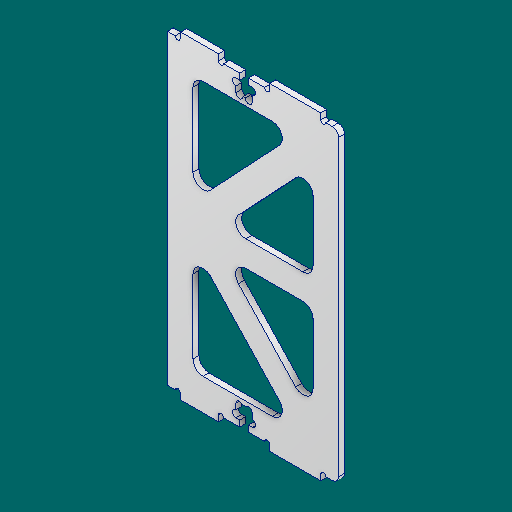
# Autodesk Inventor part: IntakeRamp
Saved by Autodesk Inventor 2023.1 (Build 271208000, 208)
## iProperties
Created: 2022-11-11
Part Number: IntakeRamp
Material: Aluminum 6061
Document SubType Name: Modeling
Designer: zac-h
Density: 2.7 g/cm^3
Appearance: Aluminum - Flat
Mass: 67.9744 g
Surface Area: 202.14 cm^2
Volume: 25.1757 cm^3
Author: zac-h
Autodesk Inventor part; units mm, degrees
ref_plane "YZ Plane" through (0, 0, 0) normal (1, 0, 0) x (0, 1, 0)
ref_plane "XZ Plane" through (0, 0, 0) normal (0, 1, 0) x (-1, 0, 0)
ref_plane "XY Plane" through (0, 0, 0) normal (0, 0, 1) x (1, 0, 0)
sketch "Sketch1" plane through (0, 0, 0) normal (0, 0, 1) x (1, 0, 0)
  line L0 (0, 0) -> (18.773541, 0)
  line L1 (18.773541, 0) -> (18.773541, 3)
  line L2 (-0.276459, 3) -> (18.773541, 3) construction
  line L3 (-0.276459, 0) -> (-0.276459, 3)
  line L4 (29.314541, 3) -> (33.632541, 3) construction
  line L5 (44.173541, 0) -> (69.573541, 0)
  line L6 (69.573541, 0) -> (69.573541, 3)
  line L7 (44.173541, 3) -> (69.573541, 3) construction
  line L8 (44.173541, 0) -> (44.173541, 3)
  line L9 (-0.276459, 3) -> (-6.626459, 3)
  line L10 (-0.276459, 3) -> (6.073541, 3) construction
  line L11 (-6.626459, 3) -> (-6.626459, 79.2)
  line L12 (-6.626459, 79.2) -> (78.463541, 79.2)
  line L13 (69.573541, 3) -> (78.463541, 3)
  line L14 (78.463541, 3) -> (78.463541, 79.2)
  line L15 (18.773541, 3) -> (29.314541, 3)
  line L16 (44.173541, 3) -> (33.632541, 3)
  line L17 (33.632541, 3) -> (33.632541, 6)
  line L18 (33.632541, 6) -> (35.537541, 6)
  line L19 (35.537541, 6) -> (35.537541, 12.35)
  line L20 (35.537541, 12.35) -> (27.409541, 12.35)
  line L21 (27.409541, 12.35) -> (27.409541, 6)
  line L22 (27.409541, 6) -> (29.314541, 6)
  line L23 (29.314541, 6) -> (29.314541, 3)
  circle A0 centre (20.023541, 3) radius 1.25
  circle A1 centre (-1.526459, 3) radius 1.25
  circle A2 centre (42.923541, 3) radius 1.25
  circle A3 centre (70.823541, 3) radius 1.25
  circle A4 centre (35.537541, 7.75) radius 1.75
  circle A5 centre (27.409541, 7.75) radius 1.75
  circle A6 centre (33.787541, 12.35) radius 1.75
  circle A7 centre (29.159541, 12.35) radius 1.75
  point P0 (28.362041, 6)
  point P1 (21.273541, 3)
  point P2 (27.409541, 9.5)
  point P3 (30.909541, 12.35)
  point P4 (32.037541, 12.35)
  point P5 (35.537541, 9.5)
  point P6 (41.673541, 3)
  point P7 (72.073541, 3)
  point P8 (-2.776459, 3)
  dimension "d9" = 2.5
  dimension "d10" = 3.5
  dimension "d11" = 3.5
  dimension "d0" = 6.35
  dimension "d1" = 180
  dimension "d2" = 76.2
  dimension "d3" = 8.89
  dimension "d4" = 3
  dimension "d5" = 8.128
  dimension "d6" = 6.35
  constraints: 30 end point, 10 point on line, 6 perpendicular, 5 horizontal, 3 collinear, 2 vertical, 1 midpoint, 1 parallel, 24 other
  measures "d0" distance of L2.start L9.end
  measures "d1" angle of L9 L10
  measures "d2" distance of L9.end L11.end
  measures "d3" distance of L6.end L13.end
  measures "d4" distance of L4.end L17.end
  measures "d5" distance between parallel lines of L19 L21
  measures "d6" distance from line of point (28.362, 6) L20
sketch "Sketch1 outline for Extrusion1" plane through (0, 0, 0) normal (0, 0, 1) x (1, 0, 0)
  line L0 (-0.276459, 3) -> (0, 0)
  arc A0 (-2.776459, 3) -> (-0.276459, 3) centre (-1.526459, 3) cw
  line L1 (-6.626459, 3) -> (-2.776459, 3)
  line L2 (-6.626459, 79.2) -> (-6.626459, 3)
  line L3 (78.463541, 79.2) -> (-6.626459, 79.2)
  line L4 (78.463541, 3) -> (78.463541, 79.2)
  line L5 (72.073541, 3) -> (78.463541, 3)
  arc A1 (69.573541, 3) -> (72.073541, 3) centre (70.823541, 3) cw
  line L6 (69.573541, 0) -> (69.573541, 3)
  line L7 (44.173541, 0) -> (69.573541, 0)
  line L8 (44.173541, 3) -> (44.173541, 0)
  arc A2 (41.673541, 3) -> (44.173541, 3) centre (42.923541, 3) cw
  line L9 (33.632541, 3) -> (41.673541, 3)
  line L10 (33.632541, 6) -> (33.632541, 3)
  line L11 (35.537541, 6) -> (33.632541, 6)
  arc A3 (35.537541, 9.5) -> (35.537541, 6) centre (35.537541, 7.75) cw
  line L12 (35.537541, 12.35) -> (35.537541, 9.5)
  arc A4 (32.037541, 12.35) -> (35.537541, 12.35) centre (33.787541, 12.35) cw
  line L13 (30.909541, 12.35) -> (32.037541, 12.35)
  arc A5 (27.409541, 12.35) -> (30.909541, 12.35) centre (29.159541, 12.35) cw
  line L14 (27.409541, 9.5) -> (27.409541, 12.35)
  arc A6 (27.409541, 6) -> (27.409541, 9.5) centre (27.409541, 7.75) cw
  line L15 (29.314541, 6) -> (27.409541, 6)
  line L16 (29.314541, 3) -> (29.314541, 6)
  line L17 (21.273541, 3) -> (29.314541, 3)
  arc A7 (18.773541, 3) -> (21.273541, 3) centre (20.023541, 3) cw
  line L18 (18.773541, 0) -> (18.773541, 3)
  line L19 (0, 0) -> (18.773541, 0)
extrude "Extrusion1" add sketch "Sketch1 outline for Extrusion1" along normal blind 3
fillet "Fillet1" radius 1.75 2 edges at (30.9095, 12.35, 1.5) (32.0375, 12.35, 1.5)
mirror "Mirror1" about plane through (78.463541, 79.2, 0) normal (0, 1, 0) of "Extrusion1"
sketch "Sketch2" plane through (0, 0, 3) normal (0, 0, 1) x (1, 0, 0)
  arc A0 (30.316541, 13.662955) -> (32.630541, 13.662955) centre (31.473541, 14.97591) ccw
  arc A1 (35.537541, 12.35) -> (32.630541, 13.662955) centre (33.787541, 12.35) ccw
  line L0 (35.537541, 12.35) -> (35.537541, 9.5)
  arc A2 (35.537541, 6) -> (35.537541, 9.5) centre (35.537541, 7.75) ccw
  line L1 (35.537541, 6) -> (33.632541, 6)
  line L2 (33.632541, 6) -> (33.632541, 3)
  line L3 (33.632541, 3) -> (41.673541, 3)
  arc A3 (44.173541, 3) -> (41.673541, 3) centre (42.923541, 3) ccw
  line L4 (44.173541, 3) -> (44.173541, 0)
  line L5 (44.173541, 0) -> (69.573541, 0)
  line L6 (69.573541, 0) -> (69.573541, 3)
  arc A4 (72.073541, 3) -> (69.573541, 3) centre (70.823541, 3) ccw
  line L7 (72.073541, 3) -> (78.463541, 3)
  line L8 (78.463541, 3) -> (78.463541, 155.4)
  line L9 (72.073541, 155.4) -> (78.463541, 155.4)
  arc A5 (69.573541, 155.4) -> (72.073541, 155.4) centre (70.823541, 155.4) ccw
  line L10 (69.573541, 158.4) -> (69.573541, 155.4)
  line L11 (44.173541, 158.4) -> (69.573541, 158.4)
  line L12 (44.173541, 155.4) -> (44.173541, 158.4)
  arc A6 (41.673541, 155.4) -> (44.173541, 155.4) centre (42.923541, 155.4) ccw
  line L13 (33.632541, 155.4) -> (41.673541, 155.4)
  line L14 (33.632541, 152.4) -> (33.632541, 155.4)
  line L15 (35.537541, 152.4) -> (33.632541, 152.4)
  arc A7 (35.537541, 148.9) -> (35.537541, 152.4) centre (35.537541, 150.65) ccw
  line L16 (35.537541, 146.05) -> (35.537541, 148.9)
  arc A8 (32.037541, 146.05) -> (35.537541, 146.05) centre (33.787541, 146.05) ccw
  line L17 (30.909541, 146.05) -> (32.037541, 146.05)
  arc A9 (27.409541, 146.05) -> (30.909541, 146.05) centre (29.159541, 146.05) ccw
  line L18 (27.409541, 148.9) -> (27.409541, 146.05)
  arc A10 (27.409541, 152.4) -> (27.409541, 148.9) centre (27.409541, 150.65) ccw
  line L19 (29.314541, 152.4) -> (27.409541, 152.4)
  line L20 (29.314541, 155.4) -> (29.314541, 152.4)
  line L21 (21.273541, 155.4) -> (29.314541, 155.4)
  arc A11 (18.773541, 155.4) -> (21.273541, 155.4) centre (20.023541, 155.4) ccw
  line L22 (18.773541, 158.4) -> (18.773541, 155.4)
  line L23 (0, 158.4) -> (18.773541, 158.4)
  line L24 (-0.276459, 155.4) -> (0, 158.4)
  arc A12 (-2.776459, 155.4) -> (-0.276459, 155.4) centre (-1.526459, 155.4) ccw
  line L25 (-6.626459, 155.4) -> (-2.776459, 155.4)
  line L26 (-6.626459, 3) -> (-6.626459, 155.4)
  line L27 (-6.626459, 3) -> (-2.776459, 3)
  arc A13 (-0.276459, 3) -> (-2.776459, 3) centre (-1.526459, 3) ccw
  line L28 (-0.276459, 3) -> (0, 0)
  line L29 (0, 0) -> (18.773541, 0)
  line L30 (18.773541, 0) -> (18.773541, 3)
  arc A14 (21.273541, 3) -> (18.773541, 3) centre (20.023541, 3) ccw
  line L31 (21.273541, 3) -> (29.314541, 3)
  line L32 (29.314541, 3) -> (29.314541, 6)
  line L33 (29.314541, 6) -> (27.409541, 6)
  arc A15 (27.409541, 9.5) -> (27.409541, 6) centre (27.409541, 7.75) ccw
  line L34 (27.409541, 9.5) -> (27.409541, 12.35)
  arc A16 (30.316541, 13.662955) -> (27.409541, 12.35) centre (29.159541, 12.35) ccw
  line L35 (6.073541, 15.7) -> (65.763541, 15.7)
  line L36 (65.763541, 15.7) -> (65.763541, 142.7)
  line L37 (65.763541, 142.7) -> (6.073541, 142.7)
  line L38 (6.073541, 142.7) -> (6.073541, 15.7)
  line L39 (6.073541, 79.2) -> (65.763541, 79.2) construction
  line L40 (6.073541, 72.85) -> (65.763541, 72.85)
  line L41 (65.763541, 85.55) -> (6.073541, 85.55)
  arc A17 (6.073541, 85.55) -> (6.073541, 72.85) centre (6.073541, 79.2) ccw
  arc A18 (65.763541, 72.85) -> (65.763541, 85.55) centre (65.763541, 79.2) ccw
  line L42 (65.763541, 142.7) -> (6.073541, 79.2) construction
  line L43 (61.136755, 147.049179) -> (1.446755, 83.549179)
  line L44 (10.700327, 74.850821) -> (70.390327, 138.350821)
  arc A19 (70.390327, 138.350821) -> (61.136755, 147.049179) centre (65.763541, 142.7) ccw
  arc A20 (1.446755, 83.549179) -> (10.700327, 74.850821) centre (6.073541, 79.2) ccw
  line L45 (65.763541, 15.7) -> (6.073541, 79.2) construction
  line L46 (70.390327, 20.049179) -> (10.700327, 83.549179)
  line L47 (1.446755, 74.850821) -> (61.136755, 11.350821)
  arc A21 (61.136755, 11.350821) -> (70.390327, 20.049179) centre (65.763541, 15.7) ccw
  arc A22 (10.700327, 83.549179) -> (1.446755, 74.850821) centre (6.073541, 79.2) ccw
  point P0 (35.918541, 79.2)
  point P1 (35.918541, 110.95)
  point P2 (35.918541, 47.45)
  point P3 (57.048527, 15.7)
  point P4 (6.073541, 69.928709)
  point P5 (20.757554, 72.85)
  point P6 (65.763541, 24.971291)
  point P7 (65.763541, 133.428709)
  point P8 (20.757554, 85.55)
  point P9 (65.763541, 85.55)
  point P10 (6.073541, 88.471291)
  point P11 (57.048527, 142.7)
  dimension "d13" = 12.7
  dimension "d14" = 12.7
  dimension "d15" = 12.7
  dimension "d16" = 12.7
  dimension "d28" = 12.7
  dimension "d29" = 12.7
  constraints: 32 end point, 12 point on circle, 12 tangent, 6 centre point, 5 midpoint, 5 parallel, 1 concentric, 1 horizontal, 1 perpendicular
  measures "d13" distance between parallel lines of L26 L38
  measures "d14" distance between parallel lines of L36 L8
  measures "d15" distance between parallel lines of L9 L37
  measures "d16" distance between parallel lines of L7 L35
  measures "d28" diameter of A18
  measures "d29" diameter of A20
extrude "Extrusion2" cut sketch "Sketch2" against normal blind 3 contours L38 L47 L35 | L46 L40 L36 | L38 L37 L43 | L44 L36 L41
fillet "Fillet2" radius 3.175 2 edges at (78.4635, 155.4, 1.5) (78.4635, 3, 1.5)
fillet "Fillet3" radius 5 12 edges at (20.7576, 72.85, 1.5) (65.7635, 72.85, 1.5) (65.7635, 24.9713, 1.5) (65.7635, 133.4287, 1.5) (65.7635, 85.55, 1.5) (20.7576, 85.55, 1.5) (57.0485, 15.7, 1.5) (6.0735, 15.7, 1.5) (6.0735, 69.9287, 1.5) (6.0735, 88.4713, 1.5) (6.0735, 142.7, 1.5) (57.0485, 142.7, 1.5)
body "Solid1"
